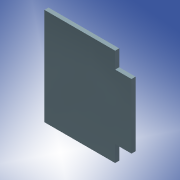
# Autodesk Inventor part: BB001
Saved by Autodesk Inventor 2017 SP1 (Build 210196100, 196)
## iProperties
Created: 2017-08-08
Part Number: BB001
Material: ABS Plastic
Document SubType Name: Modeling
Designer: Zach
Density: 1.06 g/cm^3
Appearance: CR Light Blue
Author: Zach
Autodesk Inventor part; units mm, degrees
ref_plane "YZ Plane" through (0, 0, 0) normal (1, 0, 0) x (0, 1, 0)
ref_plane "XZ Plane" through (0, 0, 0) normal (0, 1, 0) x (-1, 0, 0)
ref_plane "XY Plane" through (0, 0, 0) normal (0, 0, 1) x (1, 0, 0)
sketch "Sketch1" plane through (0, 0, 0) normal (0, 0, 1) x (1, 0, 0)
  line L0 (0, 0) -> (106.5, 0) construction
  line L1 (106.5, 0) -> (106.5, 119) construction
  line L2 (106.5, 119) -> (0, 119) construction
  line L3 (0, 119) -> (0, 0) construction
  line L4 (106.5, 119) -> (86.5, 119) construction
  line L5 (86.5, 119) -> (86.5, 99) construction
  line L6 (86.5, 99) -> (106.5, 99) construction
  line L7 (106.5, 99) -> (106.5, 119) construction
  line L8 (106.5, 0) -> (86.5, 0) construction
  line L9 (86.5, 0) -> (86.5, 20) construction
  line L10 (86.5, 20) -> (106.5, 20) construction
  line L11 (106.5, 20) -> (106.5, 0) construction
  line L12 (0, 119) -> (86.5, 119)
  line L13 (86.5, 119) -> (86.5, 99)
  line L14 (86.5, 99) -> (106.5, 99)
  line L15 (106.5, 20) -> (86.5, 20)
  line L16 (86.5, 0) -> (86.5, 20)
  line L17 (86.5, 0) -> (0, 0)
  line L18 (0, 0) -> (0, 119)
  line L19 (106.5, 99) -> (106.5, 20)
  dimension "d0" = 106.5
  dimension "d1" = 119
  dimension "d2" = 20
  dimension "d3" = 20
  dimension "d4" = 20
  dimension "d5" = 20
  constraints: 40 end point, 7 collinear, 6 parallel, 4 perpendicular, 3 horizontal
  measures "d0" distance of L2.end L1.end
  measures "d1" distance of L1.end L0.end
  measures "d2" distance of L6.end L5.end
  measures "d3" distance of L4.end L5.end
  measures "d4" distance of L9.end L10.end
  measures "d5" distance of L8.end L9.end
extrude "Extrusion1" add sketch "Sketch1" along normal blind 5
body "Solid1"
